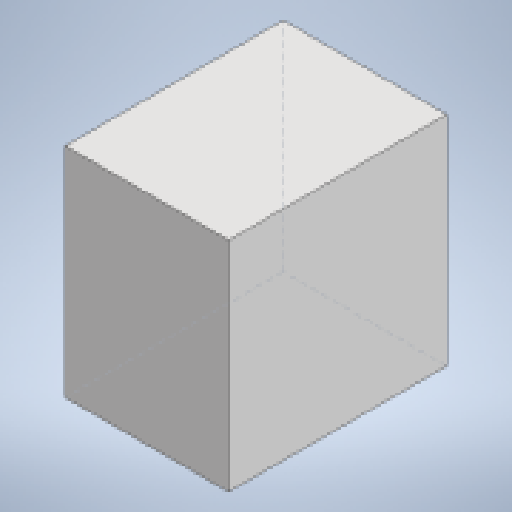
# Autodesk Inventor part: arm-right
Saved by Autodesk Inventor 2025 (Build 290162000, 162)
## iProperties
Created: 2026-01-29
Part Number: arm-right
Material: 一般
Document SubType Name: Modeling
Designer: mahhy
Density: 1 g/cm^3
Appearance: 既定
Author: mahhy
Autodesk Inventor part; units mm, degrees
ref_plane "YZ Plane" through (0, 0, 0) normal (1, 0, 0) x (0, 1, 0)
ref_plane "XZ Plane" through (0, 0, 0) normal (0, 1, 0) x (-1, 0, 0)
ref_plane "XY Plane" through (0, 0, 0) normal (0, 0, 1) x (1, 0, 0)
sketch "スケッチ1" plane through (0, 0, 0) normal (0, 1, 0) x (-1, 0, 0)
  line L0 (0, 0) -> (30, 0)
  line L1 (30, 0) -> (30, -20)
  line L2 (30, -20) -> (0, -20)
  line L3 (0, -20) -> (0, 0)
  dimension "d0" = 30
  dimension "d1" = 20
  constraints: 8 end point, 2 parallel, 1 horizontal, 1 perpendicular
  measures "d0" distance of L1.end L2.end
  measures "d1" distance of L0.end L1.end
extrude "押し出し1" add sketch "スケッチ1" along normal blind 15
sketch "スケッチ3" plane through (0, 0, 0) normal (0, -1, 0) x (1, 0, 0)
  line L0 (-25, -17.5) -> (-15, -17.5)
  line L1 (-15, -17.5) -> (-15, -2.5)
  line L2 (-15, -2.5) -> (-25, -2.5)
  line L3 (-25, -2.5) -> (-25, -17.5)
  line L4 (-30, -20) -> (-30, 0) projected
  point P0 (0, 0)
  point P1 (-25, -10)
  point P2 (-30, -10)
  dimension "d4" = 15
  dimension "d5" = 10
  dimension "d6" = 5
  constraints: 8 end point, 2 midpoint, 2 parallel, 1 horizontal, 1 horizontal alignment, 1 perpendicular
  measures "d4" distance of L2.end L0.start
  measures "d5" distance of L1.end L2.end
  measures "d6" distance between parallel lines of L4 L3
extrude "押し出し2" cut sketch "スケッチ3" against normal blind 5
sketch "スケッチ4" plane through (0, 15, 0) normal (0, 1, 0) x (1, 0, 0)
  circle A0 centre (-20, 10) radius 1.5 projected
  point P0 (0, 0)
extrude "押し出し4" cut sketch "スケッチ4" against normal through all
sketch "スケッチ5" plane through (0, 15, 0) normal (0, 1, 0) x (1, 0, 0)
  circle A0 centre (-20, 10) radius 1.5 projected
  circle A1 centre (-20, 10) radius 3.5
  point P0 (0, 0)
  dimension "d13" = 7
  constraints: 1 centre point, 1 coincident
  measures "d13" diameter of A1
extrude "押し出し5" cut sketch "スケッチ5" against normal blind 5
sketch "スケッチ6" plane through (-20, 10, -10) normal (0, 1, 0) x (1, 0, 0)
  line L0 (0, 2.6) -> (2.2517, 1.3)
  line L1 (2.2517, 1.3) -> (2.2517, -1.3)
  line L2 (2.2517, -1.3) -> (0, -2.6)
  line L3 (0, -2.6) -> (-2.2517, -1.3)
  line L4 (-2.2517, -1.3) -> (-2.2517, 1.3)
  line L5 (-2.2517, 1.3) -> (0, 2.6)
  circle A0 centre (0, 0) radius 1.5 projected
  line L6 (-10, 10) -> (-10, -10) projected
  point P0 (20, -10)
  dimension "d16" = 2.6
  constraints: 12 end point, 1 coincident, 1 parallel, 13 other
  measures "d16" distance of L3.end L4.end
extrude "押し出し6" cut sketch "スケッチ6" against normal blind 3
sketch "スケッチ7" plane through (0, 0, -20) normal (0, 0, -1) x (-1, 0, 0)
  line L0 (0, 0) -> (30, 0) projected
  line L1 (28, 2) -> (21, 2)
  line L2 (21, 2) -> (21, 37)
  line L3 (21, 37) -> (28, 37)
  line L4 (28, 37) -> (28, 2)
  line L5 (30, 0) -> (30, 15) projected
  dimension "d29" = 7
  dimension "d30" = 35
  dimension "d31" = 2
  dimension "d32" = 2
  constraints: 8 end point, 2 parallel, 1 horizontal, 1 perpendicular
  measures "d29" distance of L2.end L3.end
  measures "d30" distance of L1.end L2.end
  measures "d31" distance between parallel lines of L0 L1
  measures "d32" distance between parallel lines of L5 L4
extrude "押し出し7" add sketch "スケッチ7" along normal blind 15
sketch "スケッチ8" plane through (0, 0, -35) normal (0, 0, -1) x (-1, 0, 0)
  line L0 (28, 2) -> (28, 37) projected
  line L1 (21, 37) -> (21, 2) projected
  line L2 (28, 27) -> (21, 27)
  line L3 (21, 27) -> (21, 12)
  line L4 (21, 12) -> (28, 12)
  line L5 (28, 12) -> (28, 27)
  line L6 (21, 2) -> (28, 2) projected
  line L7 (28, 37) -> (21, 37) projected
  point P0 (0, 0)
  dimension "d33" = 15
  dimension "d34" = 10
  dimension "d35" = 10
  constraints: 8 end point, 2 parallel, 2 point on line, 1 horizontal, 1 perpendicular
  measures "d33" distance of L3.end L2.end
  measures "d34" distance between parallel lines of L6 L4
  measures "d35" distance between parallel lines of L7 L2
extrude "押し出し8" cut sketch "スケッチ8" against normal blind 8 contours L4 L1 L2 L0
move faces "移動1" translate (0, 0, -10) faces at (-20, 10, 0)
sketch "スケッチ9" plane through (-28, 15, -20) normal (-1, 0, 0) x (0, 0, 1)
  line L0 (-15, -13) -> (-15, -3) projected
  line L1 (-15, -13) -> (-13, -13)
  line L2 (-13, -13) -> (-13, -3)
  line L3 (-13, -3) -> (-15, -3)
  line L4 (-15, -3) -> (-15, -13)
  line L5 (-15, 12) -> (-7, 12) projected
  line L6 (-15, 12) -> (-13, 12)
  line L7 (-13, 12) -> (-13, 22)
  line L8 (-13, 22) -> (-15, 22)
  line L9 (-15, 22) -> (-15, 12)
  point P0 (20, -15)
  dimension "d46" = 2
  constraints: 16 end point, 4 parallel, 2 horizontal, 2 perpendicular, 1 point on line
  measures "d46" distance of L8.end L7.end
extrude "押し出し9" add sketch "スケッチ9" along normal blind 2
equation "\"d32\" = d31"
equation "\"d34\" = d35"
